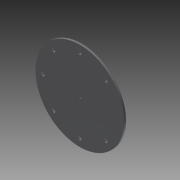
# Autodesk Inventor part: Base top
Saved by Autodesk Inventor 2015 (Build 190159000, 159)
## iProperties
Created: 2017-04-18
Part Number: Base top
Material: ABS Plastic
Document SubType Name: Modeling
Designer: Silas
Density: 1.06 g/cm^3
Appearance: Smooth - White
Author: Silas
Autodesk Inventor part; units mm, degrees
ref_plane "YZ Plane" through (0, 0, 0) normal (1, 0, 0) x (0, 1, 0)
ref_plane "XZ Plane" through (0, 0, 0) normal (0, 1, 0) x (-1, 0, 0)
ref_plane "XY Plane" through (0, 0, 0) normal (0, 0, 1) x (1, 0, 0)
sketch "Sketch1" plane through (0, 0, 0) normal (0, 1, 0) x (-1, 0, 0)
  circle A0 centre (0, 0) radius 60
  dimension "d0" = 120
  constraints: 1 centre point, 1 coincident
  measures "d0" diameter of A0
extrude "Extrusion1" add sketch "Sketch1" along normal blind 2.5
sketch "Sketch2" plane through (0, 0, 0) normal (0, 0, 1) x (1, 0, 0)
  line L0 (60, 2.5) -> (-60, 2.5) projected
  line L1 (-10, 17.5) -> (-4, 17.5)
  line L2 (10, 17.5) -> (10, 2.5)
  line L3 (10, 2.5) -> (-10, 2.5)
  line L4 (-10, 2.5) -> (-10, 17.5)
  circle A0 centre (0, 17.5) radius 10
  circle A1 centre (0, 17.5) radius 4
  line L5 (4, 17.5) -> (10, 17.5)
  line L6 (-4, 17.5) -> (4, 17.5)
  point P0 (0, 0)
  point P1 (0, 2.5)
  dimension "d3" = 20
  dimension "d4" = 15
  dimension "d5" = 8
  constraints: 12 end point, 4 parallel, 3 horizontal, 3 perpendicular, 2 centre point, 2 midpoint, 2 point on circle, 1 coincident, 1 tangent
  measures "d3" distance of L2.end L3.end
  measures "d4" distance of L2.start L2.end
  measures "d5" diameter of A1
extrude "Extrusion2" add sketch "Sketch2" along normal mid plane 18 contours L0 L4 A0 L2 | L5 A1 L1 A0 | A0 L1 A1 L5
sketch "Sketch4" plane through (10, 2.5, 9) normal (1, 0, 0) x (0, 0, -1)
  line L0 (18, 15) -> (0, 15) projected
  line L1 (18, 15) -> (18, 15) projected
  line L2 (0, 15) -> (18, 15) projected
  line L3 (0, 15) -> (0, 15) projected
  line L4 (18, 15) -> (0, 15) projected
  line L5 (0, 0) -> (0, 15) projected
  line L6 (18, 0) -> (0, 0) projected
  line L7 (18, 15) -> (18, 0) projected
  line L8 (5, 25) -> (13, 25)
  line L9 (13, 25) -> (13, 0)
  line L10 (13, 0) -> (5, 0)
  line L11 (5, 0) -> (5, 25)
  line L12 (69, 0) -> (-51, 0) projected
  point P0 (9, -2.5)
  point P1 (9, 0)
  dimension "d8" = 8
  dimension "d9" = 25
  constraints: 8 end point, 2 midpoint, 2 parallel, 1 horizontal, 1 perpendicular
  measures "d8" distance of L9.end L10.end
  measures "d9" distance of L8.end L9.end
extrude "Extrusion3" cut sketch "Sketch4" against normal blind 20 contours L9 L6 L11 L0 | L0 L11 L8 L9
sketch "Sketch5" plane through (0, 2.5, 0) normal (0, 1, 0) x (1, 0, 0)
  line L0 (10, -4) -> (10, -9) projected
  line L1 (10, -9) -> (-10, -9) projected
  line L2 (-10, -9) -> (-10, -4) projected
  line L3 (10, -4) -> (-10, -4) projected
  line L4 (10, 4) -> (-10, 4) projected
  line L5 (-10, 4) -> (-10, 9) projected
  line L6 (-10, 9) -> (10, 9) projected
  line L7 (10, 9) -> (10, 4) projected
  circle A0 centre (0, 0) radius 60 projected
  line L8 (1, 3) -> (-1, 3)
  line L9 (-1, 3) -> (-1, -3)
  line L10 (-1, -3) -> (1, -3)
  line L11 (1, -3) -> (1, 3)
  line L12 (-1, -3) -> (1, 3) construction
  line L13 (-1, 3) -> (1, -3) construction
  line L14 (0, 0) -> (50, 0) construction
  line L15 (0, 0) -> (50, 0) construction
  line L16 (0, 0) -> (35.3553, 35.3553) construction
  line L17 (0, 0) -> (50, 0) construction
  line L18 (0, 0) -> (0, 50) construction
  line L19 (0, 0) -> (50, 0) construction
  line L20 (0, 0) -> (-35.3553, 35.3553) construction
  line L21 (0, 0) -> (50, 0) construction
  line L22 (0, 0) -> (-50, 0) construction
  line L23 (0, 0) -> (50, 0) construction
  line L24 (0, 0) -> (-35.3553, -35.3553) construction
  line L25 (0, 0) -> (50, 0) construction
  line L26 (0, 0) -> (0, -50) construction
  line L27 (0, 0) -> (50, 0) construction
  line L28 (0, 0) -> (35.3553, -35.3553) construction
  line L29 (0, 0) -> (50, 0) construction
  circle A1 centre (0, -50) radius 2.1
  circle A2 centre (35.3553, -35.3553) radius 2.1
  circle A3 centre (50, 0) radius 2.1
  circle A4 centre (35.3553, 35.3553) radius 2.1
  circle A5 centre (0, 50) radius 2.1
  circle A6 centre (-35.3553, 35.3553) radius 2.1
  circle A7 centre (-50, 0) radius 2.1
  circle A8 centre (-35.3553, -35.3553) radius 2.1
  point P0 (0, 0)
  dimension "d13" = 120
  dimension "d17" = 6
  dimension "d18" = 2
  dimension "d19" = 50
  dimension "d20" = 0
  dimension "d21" = 50
  dimension "d22" = 45
  dimension "d23" = 50
  dimension "d24" = 90
  dimension "d25" = 50
  dimension "d26" = 135
  dimension "d27" = 50
  dimension "d28" = 180
  dimension "d29" = 50
  dimension "d30" = 135
  dimension "d31" = 50
  dimension "d32" = 90
  dimension "d33" = 50
  dimension "d34" = 45
  dimension "d35" = 4.2
  dimension "d36" = 4.2
  dimension "d37" = 4.2
  dimension "d38" = 4.2
  dimension "d39" = 4.2
  dimension "d40" = 4.2
  dimension "d41" = 4.2
  dimension "d42" = 4.2
  constraints: 44 end point, 10 horizontal, 9 coincident, 8 centre point, 8 equal length, 4 perpendicular, 2 midpoint, 2 parallel
  measures "d13" diameter of A0
  measures "d17" distance of L10.end L8.start
  measures "d18" distance of L9.end L10.end
  measures "d19" distance of L14.start L14.end
  measures "d20" distance between parallel lines of L14 L15
  measures "d21" distance of L14.start L16.end
  measures "d22" angle of L17 L16
  measures "d23" distance of L14.start L18.end
  measures "d24" angle of L19 L18
  measures "d25" distance of L14.start L20.end
  measures "d26" angle of L21 L20
  measures "d27" distance of L14.start L22.end
  measures "d28" angle of L22 L23
  measures "d29" distance of L14.start L24.end
  measures "d30" angle of L24 L25
  measures "d31" distance of L14.start L26.end
  measures "d32" angle of L26 L27
  measures "d33" distance of L14.start L28.end
  measures "d34" angle of L28 L29
  measures "d35" diameter of A1
  measures "d36" diameter of A2
  measures "d37" diameter of A3
  measures "d38" diameter of A4
  measures "d39" diameter of A5
  measures "d40" diameter of A6
  measures "d41" diameter of A7
  measures "d42" diameter of A8
extrude "Extrusion4" cut sketch "Sketch5" against normal blind 20 contours L11 L10 L9 L8 | A1 | A2 | A4 | A5 | A6 | A7 | A8
equation "\"d36\" = d35"
equation "\"d37\" = d36"
equation "\"d38\" = d37"
equation "\"d39\" = d38"
equation "\"d40\" = d39"
equation "\"d41\" = d40"
equation "\"d42\" = d41"
body "Solid1"
